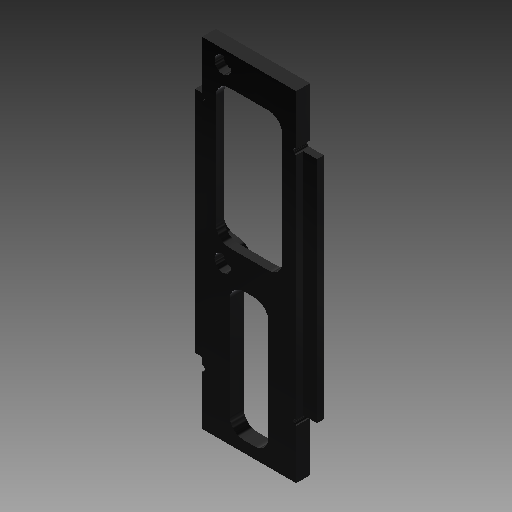
# Autodesk Inventor part: コックピット_2_サブフレーム_5
Saved by Autodesk Inventor 2018 (Build 220112000, 112)
## iProperties
Created: 2016-05-24
Part Number: コックピット_2_サブフレーム_5
Material: アセタール樹脂、黒
Document SubType Name: Modeling
Designer: hiroaki
Density: 1.425 g/cm^3
Appearance: 滑らか - 黒
Mass: 14.5233 g
Surface Area: 76.4272 cm^2
Volume: 10.1918 cm^3
Author: hiroaki
Autodesk Inventor part; units mm, degrees
ref_plane "YZ Plane" through (0, 0, 0) normal (1, 0, 0) x (0, 1, 0)
ref_plane "XZ Plane" through (0, 0, 0) normal (0, 1, 0) x (-1, 0, 0)
ref_plane "XY Plane" through (0, 0, 0) normal (0, 0, 1) x (1, 0, 0)
sketch "スケッチ1" plane through (0, 0, 0) normal (0, 0, 1) x (1, 0, 0)
  line L0 (-17, -61.25) -> (17, -61.25) construction
  line L1 (17, -61.25) -> (17, 61.25) construction
  line L2 (17, 61.25) -> (-17, 61.25) construction
  line L3 (-17, 61.25) -> (-17, -61.25) construction
  line L4 (-17, -61.25) -> (17, 61.25) construction
  line L5 (17, -61.25) -> (-17, 61.25) construction
  line L6 (-17, 43.35) -> (-17, 61.25)
  line L7 (-17, 61.25) -> (17, 61.25)
  line L8 (17, 61.25) -> (17, 43.35)
  line L9 (-17, -43.35) -> (-17, -61.25)
  line L10 (-17, -61.25) -> (17, -61.25)
  line L11 (17, -61.25) -> (17, -43.35)
  line L12 (-17, 41.25) -> (-22, 41.25)
  line L13 (-22, 41.25) -> (-22, -41.25)
  line L14 (-22, -41.25) -> (-17, -41.25)
  line L15 (17, 41.25) -> (22, 41.25)
  line L16 (22, 41.25) -> (22, -41.25)
  line L17 (22, -41.25) -> (17, -41.25)
  arc A0 (-17, 41.25) -> (-17, 43.35) centre (-17, 42.3) ccw
  arc A1 (-17, -43.35) -> (-17, -41.25) centre (-17, -42.3) ccw
  arc A2 (17, 43.35) -> (17, 41.25) centre (17, 42.3) ccw
  arc A3 (17, -41.25) -> (17, -43.35) centre (17, -42.3) ccw
  line L18 (0, 0) -> (17, 0) construction
  line L19 (0, 0) -> (0, 61.25) construction
  line L20 (-9.5, 56.25) -> (9.5, 56.25) construction
  line L21 (9.5, 56.25) -> (9.5, -5.75) construction
  line L22 (9.5, -5.75) -> (-9.5, -5.75) construction
  line L23 (-9.5, -5.75) -> (-9.5, 56.25) construction
  circle A4 centre (-9.5, 56.25) radius 1.6
  circle A5 centre (-9.5, -5.75) radius 1.6
  point P0 (0, 56.25)
  point P1 (0, 0)
  dimension "d87" = 1.05
  dimension "d88" = 122.5
  dimension "d89" = 5
  dimension "d90" = 20
  dimension "d91" = 34
  dimension "d92" = 3.2
  dimension "d93" = 7.5
  dimension "d94" = 5
  dimension "d112" = 62
  constraints: 48 end point, 10 vertical alignment, 9 perpendicular, 8 point on circle, 6 centre point, 6 midpoint, 5 horizontal, 4 collinear, 4 parallel, 4 symmetric about line, 2 coincident, 2 equal radius, 2 vertical, 1 tangent, 2 other
  measures "d87" radius of A0
  measures "d88" distance of L2.end L0.start
  measures "d89" distance between parallel lines of L13 L3
  measures "d90" distance between parallel lines of L2 L12
  measures "d91" distance of L1.end L2.end
  measures "d92" diameter of A4
  measures "d93" distance between parallel lines of L3 L23
  measures "d94" distance between parallel lines of L20 L2
  measures "d112" distance between parallel lines of L22 L20
extrude "押し出し1" add sketch "スケッチ1" along normal blind 5
sketch "スケッチ2" plane through (0, 0, 5) normal (0, 0, 1) x (1, 0, 0)
  line L0 (-17, 61.25) -> (-17, 43.35) projected
  line L1 (17, 43.35) -> (17, 61.25) projected
  line L2 (-40.5884, 60.19) -> (-17, 60.19)
  line L3 (-17, 60.19) -> (-17, -101.7483)
  line L4 (-17, -101.7483) -> (-40.5884, -101.7483)
  line L5 (-40.5884, -101.7483) -> (-40.5884, 60.19)
  line L6 (53.5752, 90.4043) -> (17, 90.4043)
  line L7 (17, 90.4043) -> (17, -93.5321)
  line L8 (17, -93.5321) -> (53.5752, -93.5321)
  line L9 (53.5752, -93.5321) -> (53.5752, 90.4043)
  point P0 (0, 0)
  constraints: 16 end point, 4 parallel, 2 collinear, 2 horizontal, 2 perpendicular
extrude "押し出し2" cut sketch "スケッチ2" against normal blind 2.5
sketch "スケッチ3" plane through (0, 0, 5) normal (0, 0, 1) x (1, 0, 0)
  line L0 (17, -41.25) -> (17, 41.25) projected
  line L1 (17, 61.25) -> (-17, 61.25) projected
  line L2 (-17, 41.25) -> (-17, -41.25) projected
  line L3 (-17, -61.25) -> (17, -61.25) projected
  circle A0 centre (-9.5, -5.75) radius 1.6 projected
  circle A1 centre (-9.5, 56.25) radius 1.6 projected
  line L4 (-7, -57.25) -> (7, -57.25)
  line L5 (7, -57.25) -> (7, -10.75)
  line L6 (7, -10.75) -> (-7, -10.75)
  line L7 (-7, -10.75) -> (-7, -57.25)
  line L8 (-12, 0.25) -> (12, 0.25)
  line L9 (12, 0.25) -> (12, 50.25)
  line L10 (12, 50.25) -> (-12, 50.25)
  line L11 (-12, 50.25) -> (-12, 0.25)
  line L12 (0, 61.25) -> (0, -61.25) construction
  line L13 (-17, 0) -> (17, 0) construction
  point P0 (0, 0)
  point P1 (0, 0.25)
  dimension "d100" = 4
  dimension "d105" = 11
  dimension "d108" = 5
  dimension "d114" = 6
  dimension "d115" = 10
  dimension "d116" = 6
  constraints: 20 end point, 5 midpoint, 4 parallel, 2 horizontal, 2 perpendicular, 1 point on line, 1 other
  measures "d100" distance between parallel lines of L3 L4
  measures "d105" distance between parallel lines of L8 L6
  measures "d108" distance between parallel lines of L2 L11
  measures "d114" distance from line of L10 A1.centre
  measures "d115" distance between parallel lines of L2 L7
  measures "d116" distance from line of L8 A0.centre
extrude "押し出し3" cut sketch "スケッチ3" against normal blind 10 contours L7 L6 L5 L4 | L11 L10 L9 L8
fillet "フィレット1" radius 5 8 edges at (-12, 50.25, 2.5) (12, 50.25, 2.5) (12, 0.25, 2.5) (-12, 0.25, 2.5) (-7, -10.75, 2.5) (-7, -57.25, 2.5) (7, -57.25, 2.5) (7, -10.75, 2.5)
sketch "スケッチ5" plane through (0, 0, 5) normal (0, 0, 1) x (1, 0, 0)
  circle A0 centre (-9.5, 56.25) radius 1.6 projected
  circle A1 centre (-9.5, -5.75) radius 1.6 projected
  circle A2 centre (-9.5, -5.75) radius 3
  circle A3 centre (-9.5, 56.25) radius 3
  point P0 (0, 0)
  dimension "d117" = 6
  dimension "d118" = 6
  constraints: 4 coincident, 2 centre point
  measures "d117" diameter of A2
  measures "d118" diameter of A3
extrude "押し出し4" cut sketch "スケッチ5" against normal blind 3.2
sketch "スケッチ6" plane through (0, 0, 0) normal (0, 0, -1) x (-1, 0, 0)
  circle A0 centre (9.5, 56.25) radius 1.6 projected
  circle A1 centre (9.5, 56.25) radius 6
  circle A2 centre (9.5, -5.75) radius 1.6 projected
  circle A3 centre (9.5, -5.75) radius 6
  line L0 (3.5, 56.25) -> (-14.5, 56.25)
  line L1 (-14.5, 56.25) -> (-14.5, -5.75)
  line L2 (-14.5, -5.75) -> (3.5, -5.75)
  line L3 (14.5, 52.9334) -> (14.5, -2.4334)
  point P0 (0, 0)
  dimension "d121" = 12
  dimension "d122" = 12
  dimension "d123" = 18
  dimension "d124" = 62
  dimension "d125" = 29
  constraints: 8 end point, 4 point on circle, 2 centre point, 2 coincident, 2 perpendicular, 1 horizontal, 1 vertical
  measures "d121" diameter of A1
  measures "d122" diameter of A3
  measures "d123" distance of L0.start L0.end
  measures "d124" distance of L0.end L1.end
  measures "d125" distance between parallel lines of L1 L3
extrude "押し出し5" cut sketch "スケッチ6" against normal blind 2 contours A1 L3 A3 L2 L1 L0
fillet "フィレット2" radius 5 6 edges at (-3.5, -5.75, 1) (-14.5, -2.4334, 1) (-14.5, 52.9334, 1) (-3.5, 56.25, 1) (14.5, -5.75, 1) (14.5, 56.25, 1)
equation "\"d88\" = d83"
equation "\"d90\" = d84"
equation "\"d83\" = 122.5"
equation "\"d84\" = 20"
